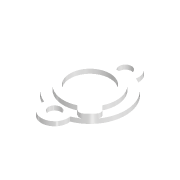
# Autodesk Inventor part: Ш.03.Створка
Saved by Autodesk Inventor 2021.3 (Build 253353010, 353A)
## iProperties
Created: 2021-07-07
Part Number: Ш.03.Створка
Material: ABS Plastic
Document SubType Name: Modeling
Designer: Михальчик
Density: 1.06 g/cm^3
Appearance: Smooth - White
Author: Михальчик
Autodesk Inventor part; units mm, degrees
ref_plane "YZ Plane" through (0, 0, 0) normal (1, 0, 0) x (0, 1, 0)
ref_plane "XZ Plane" through (0, 0, 0) normal (0, 1, 0) x (-1, 0, 0)
ref_plane "XY Plane" through (0, 0, 0) normal (0, 0, 1) x (1, 0, 0)
sketch "Sketch1" plane through (0, 0, 0) normal (0, 1, 0) x (-1, 0, 0)
  circle A0 centre (0, 0) radius 8
  circle A1 centre (0, -8) radius 3
  circle A2 centre (0, 8) radius 3
  line L0 (0, 8) -> (0, -8)
  circle A3 centre (0, 8) radius 1.4
  circle A4 centre (0, -8) radius 1.4
  line L1 (0, 11) -> (0, -11) construction
  point P0 (-2.9468, -7.4375)
  point P1 (2.9468, -7.4375)
  point P2 (2.9468, 7.4375)
  point P3 (-2.9468, 7.4375)
  dimension "d2" = 6
  dimension "d0" = 16
  dimension "d3" = 2.8
  dimension "d4" = 22
  constraints: 4 coincident, 4 end point, 3 centre point, 2 midpoint, 2 vertical, 1 equal radius, 6 other
  measures "d0" diameter of A0
  measures "d3" diameter of A3
  measures "d4" distance of L1.start L1.end
extrude "Extrusion1" add sketch "Sketch1" along normal blind 1 contours A0 A1 L0 A2 | A2 L0 A3 A0 | A0 A3 A2 | A1 A0 A4 | A0 A4 L0 A1 | L0 A1 A0 A2 | A2 A0 A3 L0 | L0 A4 A0 A1
sketch "Sketch2" plane through (0, 1, 0) normal (0, 1, 0) x (1, 0, 0)
  circle A0 centre (0, 0) radius 6
  circle A1 centre (0, 0) radius 4.5
  arc A2 (-2.9468, 7.4375) -> (-2.9468, -7.4375) centre (0, 0) ccw projected
  line L0 (-5.6569, 5.6569) -> (5.6569, -5.6569) construction
  arc A3 (2.9468, -7.4375) -> (2.9468, 7.4375) centre (0, 0) ccw projected
  line L1 (-7.0711, 4.2426) -> (4.2426, -7.0711)
  line L2 (7.0711, -4.2426) -> (-4.2426, 7.0711)
  arc A4 (-4.2426, 7.0711) -> (-7.0711, 4.2426) centre (-5.6569, 5.6569) ccw
  arc A5 (4.2426, -7.0711) -> (7.0711, -4.2426) centre (5.6569, -5.6569) ccw
  circle A6 centre (0, 8) radius 1.4 projected
  line L3 (0, 0) -> (0, 8) construction
  point P0 (5.4142, -2.5858)
  point P1 (-2.5858, 5.4142)
  point P2 (-4.063, 6.8914)
  point P3 (-6.8914, 4.063)
  point P4 (-5.4142, 2.5858)
  point P5 (2.5858, -5.4142)
  point P6 (4.063, -6.8914)
  point P7 (6.8914, -4.063)
  dimension "d7" = 12
  dimension "d8" = 9
  dimension "d9" = 4
  dimension "d10" = 45
  constraints: 10 end point, 6 point on circle, 4 centre point, 4 tangent, 3 coincident, 1 midpoint, 1 parallel, 1 vertical
  measures "d7" diameter of A0
  measures "d8" diameter of A1
  measures "d9" diameter of A5
  measures "d10" angle of L3 L0
extrude "Extrusion2" add sketch "Sketch2" along normal blind 1 contours A0 L2 A1 | L2 A1 L1 A0 | A0 L1 A2 L2 | L2 A3 L1 A0 | A0 L1 A1 L2 | L1 A1 A0
fillet "Fillet1" radius 1 4 edges at (4.063, 1.5, 6.8914) (6.8914, 1.5, 4.063) (-4.063, 1.5, -6.8914) (-6.8914, 1.5, -4.063)
body "Solid1"
